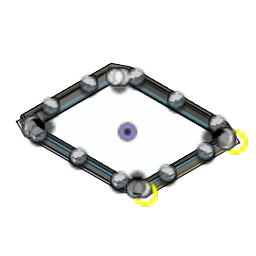
500EnclosureFusion360_Source (Autodesk Fusion 360 archive; units mm, degrees)
design "500顶盖"
Autodesk Fusion 360 part; units mm, degrees
note: some values were not read from the file. Chosen so that the rebuilt part matches the saved one: that a step has no effect; which face or edge a step refers to. Set by a fixed rule: which sketch regions a step uses.
extrude "拉伸6" [no effect]
extrude "拉伸8" [no effect]
sketch "草图4" plane through (0, 0, 31.8) normal (0, 0, 1) x (-1, 0, 0)
  line L0 (77, -57.5) -> (72, -62.5)
  line L1 (72, -62.5) -> (-71, -62.5)
  line L2 (-71, -62.5) -> (-76, -57.5)
  line L3 (-76, -57.5) -> (-76, 57.5)
  line L4 (-76, 57.5) -> (-71, 62.5)
  line L5 (-71, 62.5) -> (72, 62.5)
  line L6 (72, 62.5) -> (77, 57.5)
  line L7 (77, 57.5) -> (77, -57.5)
  line L8 (65.8, 72.5) -> (-67.2, 72.5)
  line L9 (-67.2, 72.5) -> (-87.2, 62.5)
  line L10 (-87.2, 62.5) -> (-87.2, -62.5)
  line L11 (-87.2, -62.5) -> (-67.2, -72.5)
  line L12 (-67.2, -72.5) -> (65.8, -72.5)
  line L13 (65.8, -72.5) -> (85.8, -62.5)
  line L14 (85.8, -62.5) -> (85.8, 62.5)
  line L15 (85.8, 62.5) -> (65.8, 72.5)
  circle A0 centre (-57.2, 68) radius 1.4
  circle A1 centre (-0.0001, 68) radius 1.4
  circle A2 centre (55.8, 68) radius 1.4
  circle A3 centre (80.3, 26.5) radius 1.4
  circle A4 centre (80.3, -26.5) radius 1.4
  circle A5 centre (-0.0001, -68) radius 1.4
  circle A6 centre (55.8, -68) radius 1.4
  circle A7 centre (-57.2, -68) radius 1.4
  circle A8 centre (-81.7, 26.5) radius 1.4
  circle A9 centre (-81.7, -26.5) radius 1.4
  line L16 (-87.2, -62.5) -> (-87.2, 62.5)
  line L17 (85.8, -62.5) -> (85.8, 62.5)
  line L18 (85.8, 62.5) -> (65.8, 72.5)
  line L19 (65.8, 72.5) -> (-67.2, 72.5)
  line L20 (-67.2, 72.5) -> (-87.2, 62.5)
  line L21 (-87.2, 62.5) -> (-87.2, -62.5)
  line L22 (-87.2, -62.5) -> (-67.2, -72.5)
  line L23 (-67.2, -72.5) -> (65.8, -72.5)
  line L24 (65.8, -72.5) -> (85.8, -62.5)
  line L25 (86, -62.6236) -> (86, 62.6236)
  line L26 (86, 62.6236) -> (65.8472, 72.7)
  line L27 (65.8472, 72.7) -> (-67.2472, 72.7)
  line L28 (-67.2472, 72.7) -> (-87.4, 62.6236)
  line L29 (-87.4, 62.6236) -> (-87.4, -62.6236)
  line L30 (-87.4, -62.6236) -> (-67.2472, -72.7)
  line L31 (-67.2472, -72.7) -> (65.8472, -72.7)
  line L32 (65.8472, -72.7) -> (86, -62.6236)
  line L33 (66.6262, 76) -> (-68.0262, 76)
  line L34 (-68.0262, 76) -> (-90.7, 64.6631)
  line L35 (-90.7, 64.6631) -> (-90.7, -64.6631)
  line L36 (-90.7, -64.6631) -> (-68.0262, -76)
  line L37 (-68.0262, -76) -> (66.6262, -76)
  line L38 (66.6262, -76) -> (89.3, -64.6631)
  line L39 (89.3, -64.6631) -> (89.3, 64.6631)
  line L40 (89.3, 64.6631) -> (66.6262, 76)
  line L41 (-64.8, 58.1) -> (62.2, 58.1)
  line L42 (69.2, 51.1) -> (69.2, -50.9)
  line L43 (62.2, -57.9) -> (-64.8, -57.9)
  line L44 (-71.8, -50.9) -> (-71.8, 51.1)
  arc A10 (-64.8, 58.1) -> (-71.8, 51.1) centre (-64.8, 51.1) ccw
  arc A11 (69.2, 51.1) -> (62.2, 58.1) centre (62.2, 51.1) ccw
  arc A12 (-71.8, -50.9) -> (-64.8, -57.9) centre (-64.8, -50.9) ccw
  arc A13 (62.2, -57.9) -> (69.2, -50.9) centre (62.2, -50.9) ccw
  circle A14 centre (80.3, -26.5) radius 8
  circle A15 centre (55.8, -68) radius 8
  circle A16 centre (-0.0001, -68) radius 8
  circle A17 centre (-57.2, -68) radius 8
  circle A18 centre (-81.7, -26.5) radius 8
  circle A19 centre (-81.7, 26.5) radius 8
  circle A20 centre (-57.2, 68) radius 8
  circle A21 centre (-0.0001, 68) radius 8
  circle A22 centre (55.8, 68) radius 8
  circle A23 centre (80.3, 26.5) radius 8
  circle A24 through (88.3, -26.5, 4) (76.3, -19.5718, 4) (76.3, -33.4282, 4)
  circle A25 through (63.8, -68, 4) (51.8, -61.0718, 4) (51.8, -74.9282, 4)
  circle A26 through (7.9999, -68, 4) (-4.0001, -61.0718, 4) (-4.0001, -74.9282, 4)
  circle A27 through (-49.2, -68, 4) (-61.2, -61.0718, 4) (-61.2, -74.9282, 4)
  circle A28 through (-73.7, -26.5, 4) (-85.7, -19.5718, 4) (-85.7, -33.4282, 4)
  circle A29 through (-73.7, 26.5, 4) (-85.7, 33.4282, 4) (-85.7, 19.5718, 4)
  circle A30 through (-49.2, 68, 4) (-61.2, 74.9282, 4) (-61.2, 61.0718, 4)
  circle A31 through (7.9999, 68, 4) (-4.0001, 74.9282, 4) (-4.0001, 61.0718, 4)
  circle A32 through (63.8, 68, 4) (51.8, 74.9282, 4) (51.8, 61.0718, 4)
  circle A33 through (88.3, 26.5, 4) (76.3, 33.4282, 4) (76.3, 19.5718, 4)
  line L45 (-77.9397, 57.3093) -> (-73.2093, 62.0397)
  line L46 (-73.2093, 62.0397) -> (69.4093, 62.0397)
  line L47 (69.4093, 62.0397) -> (74.1397, 57.3093)
  line L48 (74.1397, 57.3093) -> (74.1397, -57.3093)
  line L49 (74.1397, -57.3093) -> (69.4093, -62.0397)
  line L50 (69.4093, -62.0397) -> (-73.2093, -62.0397)
  line L51 (-73.2093, -62.0397) -> (-77.9397, -57.3093)
  line L52 (-77.9397, -57.3093) -> (-77.9397, 57.3093)
  line L53 (-79.3981, 57.9134) -> (-73.8134, 63.4981)
  line L54 (-73.8134, 63.4981) -> (70.0134, 63.4981)
  line L55 (70.0134, 63.4981) -> (75.5981, 57.9134)
  line L56 (75.5981, 57.9134) -> (75.5981, -57.9134)
  line L57 (75.5981, -57.9134) -> (70.0134, -63.4981)
  line L58 (70.0134, -63.4981) -> (-73.8134, -63.4981)
  line L59 (-73.8134, -63.4981) -> (-79.3981, -57.9134)
  line L60 (-79.3981, -57.9134) -> (-79.3981, 57.9134)
  point P0 (-71.8, 58.1)
  point P1 (69.2, 58.1)
  point P2 (-71.8, -57.9)
  dimension "d111" = 2.8
  dimension "d112" = 2.8
  dimension "d113" = 2.8
  dimension "d114" = 2.8
  dimension "d115" = 2.8
  dimension "d116" = 2.8
  dimension "d117" = 2.8
  dimension "d118" = 2.8
  dimension "d119" = 2.8
  dimension "d120" = 2.8
  dimension "d121" = 0.0001
  dimension "d122" = 4.5
  dimension "d123" = 30
  dimension "d124" = 4.5
  dimension "d125" = 5.5
  dimension "d126" = 46
  dimension "d127" = 5.5
  dimension "d128" = 46
  dimension "d129" = 30
  dimension "d130" = 4.5
  dimension "d131" = 4.5
  dimension "d132" = 0.0001
  dimension "d133" = 4.5
  dimension "d134" = 30
  dimension "d135" = 46
  dimension "d136" = 5.5
  dimension "d137" = 5.5
  dimension "d138" = 46
  dimension "d139" = 30
  dimension "d140" = 4.5
  dimension "d165" = 0
  dimension "d166" = 0.2
  dimension "d167" = 3.5
  dimension "d168" = 141
  dimension "d169" = 116
  dimension "d170" = 7
  dimension "d171" = 7
  dimension "d172" = 7
  dimension "d173" = 7
  dimension "d174" = 71.8
  dimension "d175" = 58.1
  dimension "d190" = 16
  dimension "d191" = 16
  dimension "d192" = 16
  dimension "d193" = 16
  dimension "d194" = 16
  dimension "d195" = 16
  dimension "d196" = 16
  dimension "d197" = 16
  dimension "d198" = 16
  dimension "d199" = 16
  dimension "d200" = 16
  dimension "d201" = 16
  dimension "d202" = 16
  dimension "d203" = 16
  dimension "d204" = 16
  dimension "d205" = 16
  dimension "d206" = 16
  dimension "d207" = 16
  dimension "d208" = 16
  dimension "d209" = 16
  constraint horizontal L41
  constraint vertical L42
  constraint horizontal L43
  constraint vertical L44
  constraint coincident P0 L41
  constraint coincident P0 L44
  constraint tangent L41 A10
  constraint tangent L44 A10
  constraint coincident P1 L41
  constraint coincident P1 L42
  constraint tangent L41 A11
  constraint tangent L42 A11
  constraint coincident P2 L43
  constraint coincident P2 L44
  constraint tangent L43 A12
  constraint tangent L44 A12
  constraint tangent L42 A13
  constraint tangent L43 A13
  constraint concentric A4 A14
  constraint concentric A6 A15
  constraint concentric A5 A16
  constraint concentric A7 A17
  constraint concentric A9 A18
  constraint concentric A8 A19
  constraint concentric A0 A20
  constraint concentric A1 A21
  constraint concentric A2 A22
  constraint concentric A3 A23
  measures "d111" diameter of A0
  measures "d112" diameter of A1
  measures "d113" diameter of A2
  measures "d114" diameter of A3
  measures "d115" diameter of A4
  measures "d116" diameter of A5
  measures "d117" diameter of A6
  measures "d118" diameter of A7
  measures "d119" diameter of A8
  measures "d120" diameter of A9
  measures "d121" horizontal distance of origin A1.centre
  measures "d122" distance of L8 A1.centre
  measures "d123" distance of L14 A2.centre
  measures "d124" distance of L8 A2.centre
  measures "d125" distance of L14 A3.centre
  measures "d126" distance of L8 A3.centre
  measures "d127" distance of L14 A4.centre
  measures "d128" distance of L12 A4.centre
  measures "d129" distance of L14 A6.centre
  measures "d130" distance of L12 A6.centre
  measures "d131" distance of L12 A5.centre
  measures "d132" horizontal distance of origin A5.centre
  measures "d133" distance of L12 A7.centre
  measures "d134" distance of A7.centre L16
  measures "d135" distance of L12 A9.centre
  measures "d136" distance of L10 A9.centre
  measures "d137" distance of L10 A8.centre
  measures "d138" distance of L8 A8.centre
  measures "d139" distance of L10 A0.centre
  measures "d140" distance of L8 A0.centre
  measures "d165" distance of L12
  measures "d168" distance of P0 P1
  measures "d169" distance of P0 P2
  measures "d170" radius of A10
  measures "d171" radius of A11
  measures "d172" radius of A12
  measures "d173" radius of A13
  measures "d174" distance of origin L44
  measures "d175" distance of origin L41
  measures "d190" diameter of A14
  measures "d191" diameter of A15
  measures "d192" diameter of A16
  measures "d193" diameter of A17
  measures "d194" diameter of A18
  measures "d195" diameter of A19
  measures "d196" diameter of A20
  measures "d197" diameter of A21
  measures "d198" diameter of A22
  measures "d199" diameter of A23
extrude "拉伸16" add sketch "草图4" along normal blind 10 contours L0 L1 L7 L12 L13 L14 L17 L23 L24 A14 A15 L57 L58 | L0 L1 L7 A14 L56 L57 | L7 A14 L56 | L7 L14 L17 A14 | L1 A15 L57 L58 | L1 A14 A15 L48 L49 L50 L56 L57 | L7 A14 A23 L56 | L7 L14 L17 A14 A23 | A14 L48 L56 | L1 A15 L58 | L1 A15 L50 | L7 A23 L56 | L7 L14 L17 A23 | A14 A23 L48 L56 | L2 L3 L4 A14 A15 A16 A17 A18 A19 A20 A21 A22 A23 L46 L47 L48 L49 L50 | A14 L48 | L1 A15 A16 L58 | L1 A15 A16 L50 | L12 L23 A15 L58 | A15 L50 | L5 L6 L7 A23 L55 L56 | L5 L6 L7 L8 L14 L15 L17 L18 L19 A22 A23 L54 L55 | A23 L48 L56 | L1 A16 L58 | L1 A16 L50 | L12 L23 A15 A16 L58 | L5 A22 A23 L46 L47 L48 L55 L56 | A23 L48 | L1 A16 A17 L58 | L1 A16 A17 L50 | L12 L23 A16 L58 | A16 L50 | L1 A17 L58 | L1 A17 L50 | L12 L23 A16 A17 L58 | L5 A22 L54 L55 | L1 L2 A17 A18 L50 L51 L52 L58 L59 L60 | L1 L2 A17 L50 | L12 L23 A17 L58 | A17 L50 | L5 A22 L46 | L5 A22 L54 | L8 L19 A22 L54 | L10 L11 L12 L16 L21 L22 L23 A17 A18 L58 L59 L60 | L5 A21 A22 L46 | L5 A21 A22 L54 | A22 L46 | L8 L19 A21 A22 L54 | L2 L3 A18 L50 L51 L52 | L5 A21 L46 | L5 A21 L54 | L8 L19 A21 L54 | L5 A20 A21 L46 | L5 A20 A21 L54 | A21 L46 | L8 L19 A20 A21 L54 | L3 A18 L52 | L3 A18 | A18 L52 L60 | L10 L16 L21 A18 L60 | L5 A20 L46 | L5 A20 L54 | L8 L19 A20 L54 | L3 A18 A19 L52 | A18 A19 L52 L60 | L10 L16 L21 A18 A19 L60 | L4 L5 A20 L46 | L4 L5 A19 A20 L45 L46 L52 L53 L54 L60 | A20 L46 | L8 L9 L10 L16 L19 L20 L21 A19 A20 L53 L54 L60 | L3 A19 L52 | L3 A19 | A19 L52 L60 | L10 L16 L21 A19 L60 | L3 L4 A19 L45 L46 L52
chamfer "倒角7" distance 2 distance2 2 8 edges at (87.2, 0, 41.8) (77.2, 67.5, 41.8) (0.7, 72.5, 41.8) (-75.8, 67.5, 41.8) (-85.8, 0, 41.8) (-75.8, -67.5, 41.8) (0.7, -72.5, 41.8) (77.2, -67.5, 41.8) measured on face at (-80.2667, 48.5698, 41.8) measured on face at (-80.2667, 48.5698, 41.8) measured on face at (-80.2667, 48.5698, 41.8) measured on face at (-80.2667, 48.5698, 41.8) measured on face at (-80.2667, 48.5698, 41.8) measured on face at (-80.2667, 48.5698, 41.8) measured on face at (-80.2667, 48.5698, 41.8) measured on face at (-80.2667, 48.5698, 41.8)
chamfer "倒角8" distance 8 distance2 9.6 8 edges at (71.8, -0.1, 41.8) (69.7497, -56.0497, 41.8) (1.3, -58.1, 41.8) (-67.1497, -56.0497, 41.8) (-69.2, -0.1, 41.8) (-67.1497, 55.8497, 41.8) (1.3, 57.9, 41.8) (69.7497, 55.8497, 41.8) measured on face at (-77.9109, -46.7318, 41.8) measured on face at (-77.9109, -46.7318, 41.8) measured on face at (-77.9109, -46.7318, 41.8) measured on face at (-77.9109, -46.7318, 41.8) measured on face at (-77.9109, -46.7318, 41.8) measured on face at (-77.9109, -46.7318, 41.8) measured on face at (-77.9109, -46.7318, 41.8) measured on face at (-77.9109, -46.7318, 41.8)
sketch "草图4 (curves 4 mm off its plane)" plane through (0, 0, 35.8) normal (0, 0, 1) x (-1, 0, 0)
  circle A0 centre (80.3, -26.5) radius 8
  circle A1 centre (55.8, -68) radius 8
  circle A2 centre (-0.0001, -68) radius 8
  circle A3 centre (-57.2, -68) radius 8
  circle A4 centre (-81.7, -26.5) radius 8
  circle A5 centre (-81.7, 26.5) radius 8
  circle A6 centre (-57.2, 68) radius 8
  circle A7 centre (-0.0001, 68) radius 8
  circle A8 centre (55.8, 68) radius 8
  circle A9 centre (80.3, 26.5) radius 8
extrude "拉伸17" cut sketch "草图4 (curves 4 mm off its plane)" along normal blind 20
extrude "拉伸18" cut sketch "草图4" along normal blind 2.8 contours L1 A15 L57 L58 | L1 A14 A15 L48 L49 L50 L56 L57 | A14 L48 L56 | L1 A15 L58 | L1 A15 L50 | A14 A23 L48 L56 | L1 A15 A16 L58 | L1 A15 A16 L50 | A23 L48 L56 | L1 A16 L58 | L1 A16 L50 | L5 A22 A23 L46 L47 L48 L55 L56 | L1 A16 A17 L58 | L1 A16 A17 L50 | L1 A17 L58 | L1 A17 L50 | L5 A22 L54 L55 | L1 L2 A17 A18 L50 L51 L52 L58 L59 L60 | L1 L2 A17 L50 | L5 A22 L46 | L5 A22 L54 | L5 A21 A22 L46 | L5 A21 A22 L54 | L5 A21 L46 | L5 A21 L54 | L5 A20 A21 L46 | L5 A20 A21 L54 | A18 L52 L60 | L5 A20 L46 | L5 A20 L54 | A18 A19 L52 L60 | L4 L5 A20 L46 | L4 L5 A19 A20 L45 L46 L52 L53 L54 L60 | A19 L52 L60
equation "d103 = 5 mm"
equation "d104 = d103"
equation "d105 = 5 mm"
equation "d106 = d105"
equation "d107 = 5 mm"
equation "d108 = d107"
equation "d109 = 5 mm"
equation "d110 = d109"
